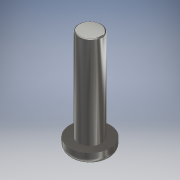
# Autodesk Inventor part: M2
Saved by Autodesk Inventor 2017 (Build 210142000, 142)
## iProperties
Created: 2019-12-06
Part Number: M2
Material: Generic
Document SubType Name: Modeling
Designer: User
Density: 1 g/cm^3
Appearance: Default
Mass: 0.0330191 g
Surface Area: 0.81068 cm^2
Volume: 0.0330191 cm^3
Author: User
Autodesk Inventor part; units mm, degrees
ref_plane "YZ Plane" through (0, 0, 0) normal (1, 0, 0) x (0, 1, 0)
ref_plane "XZ Plane" through (0, 0, 0) normal (0, 1, 0) x (-1, 0, 0)
ref_plane "XY Plane" through (0, 0, 0) normal (0, 0, 1) x (1, 0, 0)
sketch "Sketch1" plane through (0, 0, 0) normal (0, 0, 1) x (1, 0, 0)
  circle A0 centre (0, 0) radius 1
  dimension "d0" = 2
  constraints: 1 centre point, 1 coincident
  measures "d0" diameter of A0
extrude "Extrusion1" add sketch "Sketch1" along normal blind 8
sketch "Sketch2" plane through (0, 0, 0) normal (0, 0, -1) x (-1, 0, 0)
  circle A0 centre (0, 0) radius 1.75
  dimension "d3" = 3.5
  constraints: 1 centre point, 1 coincident
  measures "d3" diameter of A0
extrude "Extrusion2" add sketch "Sketch2" along normal blind 1
sketch "Sketch3" plane through (0, 0, -1) normal (0, 0, -1) x (-1, 0, 0)
  circle A0 centre (0, 0) radius 1 projected
  line L0 (-0.2879, -0.9577) -> (0.2879, -0.9577)
  line L1 (0.2879, -0.9577) -> (0.2879, 0.9577)
  line L2 (0.2879, 0.9577) -> (-0.2879, 0.9577)
  line L3 (-0.2879, 0.9577) -> (-0.2879, -0.9577)
  line L4 (-0.2879, -0.9577) -> (0.2879, 0.9577) construction
  line L5 (0.2879, -0.9577) -> (-0.2879, 0.9577) construction
  line L6 (-0.9577, 0.2879) -> (0.9577, 0.2879)
  line L7 (0.9577, 0.2879) -> (0.9577, -0.2879)
  line L8 (0.9577, -0.2879) -> (-0.9577, -0.2879)
  line L9 (-0.9577, -0.2879) -> (-0.9577, 0.2879)
  line L10 (-0.9577, 0.2879) -> (0.9577, -0.2879) construction
  line L11 (0.9577, 0.2879) -> (-0.9577, -0.2879) construction
  constraints: 24 end point, 4 midpoint, 4 parallel, 2 horizontal, 2 perpendicular, 2 point on circle
extrude "Extrusion3" cut sketch "Sketch3" against normal blind 0.5 contours L7 L8 L1 L6 | L1 L6 L3 L2 | L1 L8 L3 L6 | L0 L3 L8 L1 | L3 L8 L9 L6
fillet "Fillet1" radius 0.6 1 edges at (1.75, 0, -1)
fillet "Fillet2" radius 0.1 1 edges at (-1, 0, 8)
body "Solid1"
